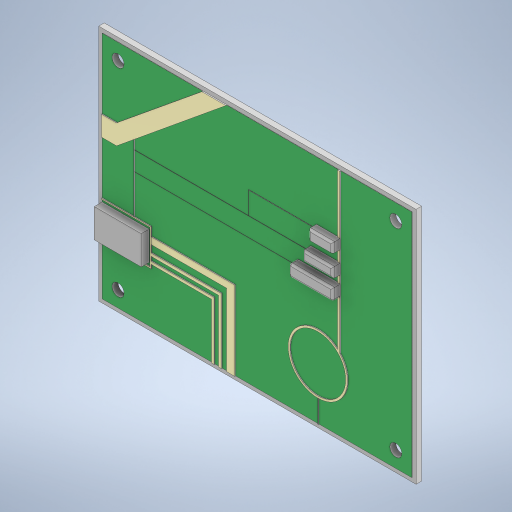
# Autodesk Inventor part: Board
Saved by Autodesk Inventor 2023 (Build 270158000, 158)
## iProperties
Created: 2022-11-08
Part Number: Board
Material: Generic
Document SubType Name: Modeling
Designer: 223076749
Density: 1 g/cm^3
Appearance: Default
Author: 223076749
Autodesk Inventor part; units mm, degrees
ref_plane "YZ Plane" through (0, 0, 0) normal (1, 0, 0) x (0, 1, 0)
ref_plane "XZ Plane" through (0, 0, 0) normal (0, 1, 0) x (-1, 0, 0)
ref_plane "XY Plane" through (0, 0, 0) normal (0, 0, 1) x (1, 0, 0)
sketch "Sketch1" plane through (0, 0, 0) normal (0, 0, 1) x (1, 0, 0)
  line L0 (0, 0) -> (203.2, 0)
  line L1 (203.2, 0) -> (203.2, 152.4)
  line L2 (203.2, 152.4) -> (0, 152.4)
  line L3 (0, 152.4) -> (0, 0)
  dimension "d0" = 203.2
  dimension "d1" = 152.4
  constraints: 8 end point, 2 parallel, 1 horizontal, 1 perpendicular
  measures "d0" distance of L2.end L1.end
  measures "d1" distance of L1.end L0.end
sketch "Sketch1 outline for Extrusion1" plane through (0, 0, 0) normal (0, 0, 1) x (1, 0, 0)
  line L0 (0, 0) -> (203.2, 0)
  line L1 (0, 152.4) -> (0, 0)
  line L2 (203.2, 152.4) -> (0, 152.4)
  line L3 (203.2, 0) -> (203.2, 152.4)
extrude "Extrusion1" add sketch "Sketch1 outline for Extrusion1" along normal blind 2.54
sketch "Sketch2" plane through (0, 0, 0) normal (0, 0, -1) x (-1, 0, 0)
  point P0 (0, 0)
sketch "Sketch4" plane through (0, 0, 2.54) normal (0, 0, 1) x (1, 0, 0)
  line L0 (0, 0) -> (203.2, 0) projected
  line L1 (101.6, 2.54) -> (200.66, 2.54)
  line L2 (200.66, 2.54) -> (200.66, 76.2)
  line L3 (2.54, 76.2) -> (2.54, 149.86)
  line L4 (0, 152.4) -> (0, 0) projected
  line L5 (2.54, 149.86) -> (101.6, 149.86)
  line L6 (203.2, 152.4) -> (0, 152.4) projected
  line L7 (200.66, 149.86) -> (101.6, 149.86)
  line L8 (203.2, 0) -> (203.2, 152.4) projected
  line L9 (200.66, 149.86) -> (200.66, 76.2)
  line L10 (2.54, 76.2) -> (2.54, 2.54)
  line L11 (2.54, 2.54) -> (101.6, 2.54)
  constraints: 16 end point, 4 perpendicular, 2 parallel, 2 point on line, 1 vertical
sketch "Sketch4 outline for Extrusion3" plane through (0, 0, 2.54) normal (0, 0, 1) x (1, 0, 0)
  line L0 (2.54, 76.2) -> (2.54, 2.54)
  line L1 (2.54, 149.86) -> (2.54, 76.2)
  line L2 (101.6, 149.86) -> (2.54, 149.86)
  line L3 (200.66, 149.86) -> (101.6, 149.86)
  line L4 (200.66, 76.2) -> (200.66, 149.86)
  line L5 (200.66, 2.54) -> (200.66, 76.2)
  line L6 (101.6, 2.54) -> (200.66, 2.54)
  line L7 (2.54, 2.54) -> (101.6, 2.54)
extrude "Extrusion3" add sketch "Sketch4 outline for Extrusion3" along normal blind 1.27
sketch "Sketch5" plane through (0, 0, 2.54) normal (0, 0, 1) x (1, 0, 0)
  line L0 (0, 0) -> (203.2, 0)
  line L1 (203.2, 0) -> (203.2, 152.4)
  line L2 (203.2, 152.4) -> (0, 152.4)
  line L3 (0, 152.4) -> (0, 0)
  line L4 (2.54, 149.86) -> (2.54, 2.54) projected
  line L5 (200.66, 149.86) -> (2.54, 149.86) projected
  line L6 (2.54, 2.54) -> (200.66, 2.54)
  line L7 (200.66, 2.54) -> (200.66, 149.86)
  line L8 (200.66, 149.86) -> (2.54, 149.86)
  line L9 (2.54, 149.86) -> (2.54, 2.54)
  constraints: 16 end point, 4 parallel, 2 horizontal, 2 perpendicular
sketch "Sketch5 outline for Extrusion4" plane through (0, 0, 2.54) normal (0, 0, 1) x (1, 0, 0)
  line L0 (0, 0) -> (203.2, 0)
  line L1 (0, 152.4) -> (0, 0)
  line L2 (203.2, 152.4) -> (0, 152.4)
  line L3 (203.2, 0) -> (203.2, 152.4)
extrude "Extrusion4" add sketch "Sketch5 outline for Extrusion4" along normal blind 1.016
sketch "Sketch6" plane through (0, 0, 3.81) normal (0, 0, 1) x (1, 0, 0)
  line L0 (0, 0) -> (12.7, 0)
  line L1 (12.7, 0) -> (12.7, 12.7)
  line L2 (12.7, 12.7) -> (0, 12.7)
  line L3 (0, 12.7) -> (0, 0)
  line L4 (203.2, 0) -> (190.5, 0)
  line L5 (190.5, 0) -> (190.5, 12.7)
  line L6 (190.5, 12.7) -> (203.2, 12.7)
  line L7 (203.2, 12.7) -> (203.2, 0)
  line L8 (203.2, 133.35) -> (203.2, 152.4)
  circle A0 centre (12.7, 12.7) radius 3.81
  circle A1 centre (190.5, 12.7) radius 3.81
  line L9 (203.2, 152.4) -> (0, 152.4) projected
  line L10 (0, 152.4) -> (12.7, 152.4)
  line L11 (12.7, 152.4) -> (12.7, 139.7)
  line L12 (12.7, 139.7) -> (0, 139.7)
  line L13 (0, 139.7) -> (0, 152.4)
  line L14 (203.2, 152.4) -> (190.5, 152.4)
  line L15 (190.5, 152.4) -> (190.5, 139.7)
  line L16 (190.5, 139.7) -> (203.2, 139.7)
  line L17 (203.2, 139.7) -> (203.2, 152.4)
  circle A2 centre (12.7, 139.7) radius 3.81
  circle A3 centre (190.5, 139.7) radius 3.81
  dimension "d18" = 12.7
  dimension "d19" = 12.7
  dimension "d21" = 12.7
  dimension "d22" = 12.7
  dimension "d28" = 7.62
  dimension "d29" = 7.62
  dimension "d30" = 12.7
  dimension "d31" = 12.7
  dimension "d32" = 12.7
  dimension "d33" = 12.7
  dimension "d34" = 7.62
  dimension "d35" = 7.62
  constraints: 34 end point, 8 parallel, 4 centre point, 4 coincident, 4 horizontal, 4 perpendicular
  measures "d18" distance of L2.end L1.end
  measures "d19" distance of L1.end L0.end
  measures "d21" distance of L5.end L6.end
  measures "d22" distance of L4.end L5.end
  measures "d28" diameter of A0
  measures "d29" diameter of A1
  measures "d30" distance of L11.end L12.end
  measures "d31" distance of L10.end L11.end
  measures "d32" distance of L16.end L15.end
  measures "d33" distance of L15.end L14.end
  measures "d34" diameter of A2
  measures "d35" diameter of A3
hole "Hole1" at (12.7, 139.7, 3.81) at (190.5, 139.7, 3.81) at (190.5, 12.7, 3.81) at (12.7, 12.7, 3.81) direction (0, 0, -1) diameter 7.62 end through all
sketch "Sketch7" plane through (0, 0, 3.81) normal (0, 0, 1) x (1, 0, 0)
  line L0 (2.54, 149.86) -> (2.54, 2.54)
  line L1 (2.54, 58.728997) -> (34.300412, 58.728997)
  line L2 (34.300412, 58.728997) -> (34.300412, 35.304324)
  line L3 (34.300412, 35.304324) -> (2.54, 35.304324)
  line L4 (2.54, 105.243705) -> (12.214291, 105.243705)
  line L5 (2.54, 98.870342) -> (12.214291, 98.870342)
  line L6 (12.214291, 98.870342) -> (73.177483, 148.650773)
  line L7 (12.214291, 92.520342) -> (2.54, 92.520342)
  line L8 (12.214291, 92.520342) -> (80.736552, 148.650773)
  line L9 (12.214291, 105.243705) -> (66.853266, 149.86)
  line L10 (200.66, 149.86) -> (2.54, 149.86)
  line L11 (73.177483, 148.650773) -> (74.658352, 149.86)
  line L12 (80.736552, 148.650773) -> (82.217421, 149.86)
  line L13 (2.54, 58.00717) -> (33.558011, 58.00717)
  line L14 (33.558011, 58.00717) -> (33.558011, 36.134305)
  line L15 (33.558011, 36.134305) -> (2.54, 36.134305)
  line L16 (2.54, 36.134305) -> (2.54, 58.00717)
  line L17 (2.54, 36.134305) -> (2.54, 35.304324)
  line L18 (2.54, 58.728997) -> (2.54, 58.00717)
  circle A0 centre (141.039906, 36.134305) radius 19.037306
  circle A1 centre (141.039906, 36.134305) radius 17.824973
  line L19 (138.373756, 98.870342) -> (158.864879, 98.870342)
  line L20 (158.864879, 98.870342) -> (158.864879, 92.520342)
  line L21 (158.864879, 92.520342) -> (138.373756, 92.520342)
  line L22 (138.373756, 92.520342) -> (138.373756, 98.870342)
  line L23 (138.373756, 112.547156) -> (158.864879, 112.547156)
  line L24 (158.864879, 112.547156) -> (158.864879, 106.496625)
  line L25 (158.864879, 106.496625) -> (138.373756, 106.496625)
  line L26 (138.373756, 106.496625) -> (138.373756, 112.547156)
  line L27 (158.864879, 87.286033) -> (151.567129, 87.286033)
  line L28 (151.567129, 87.286033) -> (151.567129, 83.13993)
  line L29 (151.567129, 83.13993) -> (158.864879, 83.13993)
  line L30 (158.864879, 83.13993) -> (158.864879, 87.286033)
  line L31 (155.216004, 149.86) -> (155.216004, 112.547156)
  line L32 (153.719902, 149.86) -> (153.719902, 112.547156)
  line L33 (153.719902, 106.496625) -> (153.719902, 98.870342)
  line L34 (155.216004, 106.496625) -> (155.216004, 98.870342)
  line L35 (153.719902, 92.520342) -> (153.719902, 87.286033)
  line L36 (155.216004, 92.520342) -> (155.216004, 87.286033)
  line L37 (153.719902, 149.86) -> (155.216004, 149.86)
  line L38 (200.66, 149.86) -> (2.54, 149.86)
  line L39 (153.719902, 112.547156) -> (155.216004, 112.547156)
  line L40 (2.54, 105.243705) -> (2.54, 92.520342)
  line L41 (66.853266, 149.86) -> (82.217421, 149.86)
  point P0 (0, 0)
  constraints: 78 end point, 27 point on line, 9 parallel, 9 perpendicular, 7 horizontal, 5 collinear, 2 centre point, 1 coincident, 1 midpoint, 1 vertical
sketch "Sketch7 outline for Extrusion6" plane through (0, 0, 3.81) normal (0, 0, 1) x (1, 0, 0)
  circle A0 centre (141.039906, 36.134305) radius 19.037306
  circle A1 centre (141.039906, 36.134305) radius 17.824973
  line L0 (34.300412, 35.304324) -> (34.300412, 58.728997)
  line L1 (2.54, 35.304324) -> (34.300412, 35.304324)
  line L2 (2.54, 36.134305) -> (2.54, 35.304324)
  line L3 (33.558011, 36.134305) -> (2.54, 36.134305)
  line L4 (33.558011, 58.00717) -> (33.558011, 36.134305)
  line L5 (2.54, 58.00717) -> (33.558011, 58.00717)
  line L6 (2.54, 58.728997) -> (2.54, 58.00717)
  line L7 (34.300412, 58.728997) -> (2.54, 58.728997)
  line L8 (82.217421, 149.86) -> (66.853266, 149.86)
  line L9 (80.736552, 148.650773) -> (82.217421, 149.86)
  line L10 (12.214291, 92.520342) -> (80.736552, 148.650773)
  line L11 (2.54, 92.520342) -> (12.214291, 92.520342)
  line L12 (2.54, 105.243705) -> (2.54, 92.520342)
  line L13 (12.214291, 105.243705) -> (2.54, 105.243705)
  line L14 (66.853266, 149.86) -> (12.214291, 105.243705)
  line L15 (155.216004, 87.286033) -> (155.216004, 92.520342)
  line L16 (153.719902, 87.286033) -> (155.216004, 87.286033)
  line L17 (153.719902, 92.520342) -> (153.719902, 87.286033)
  line L18 (155.216004, 92.520342) -> (153.719902, 92.520342)
  line L19 (155.216004, 98.870342) -> (155.216004, 106.496625)
  line L20 (153.719902, 98.870342) -> (155.216004, 98.870342)
  line L21 (153.719902, 106.496625) -> (153.719902, 98.870342)
  line L22 (155.216004, 106.496625) -> (153.719902, 106.496625)
  line L23 (153.719902, 149.86) -> (153.719902, 112.547156)
  line L24 (155.216004, 149.86) -> (153.719902, 149.86)
  line L25 (155.216004, 112.547156) -> (155.216004, 149.86)
  line L26 (153.719902, 112.547156) -> (155.216004, 112.547156)
extrude "Extrusion6" add sketch "Sketch7 outline for Extrusion6" along normal blind 0.508
sketch "Sketch9" plane through (0, 0, 3.81) normal (0, 0, 1) x (1, 0, 0)
  line L0 (155.216004, 112.547156) -> (155.216004, 149.86)
  line L1 (155.216004, 112.547156) -> (139.716798, 112.547156)
  line L2 (139.716798, 112.547156) -> (139.716798, 106.444154)
  line L3 (139.716798, 106.444154) -> (155.216004, 106.444154)
  line L4 (155.216004, 106.444154) -> (155.216004, 112.547156)
  line L5 (153.719902, 98.870342) -> (155.216004, 98.870342)
  line L6 (155.216004, 98.870342) -> (136.133648, 98.870342)
  line L7 (136.133648, 98.870342) -> (136.133648, 92.469871)
  line L8 (136.133648, 92.469871) -> (155.216004, 92.469871)
  line L9 (155.216004, 92.469871) -> (155.216004, 98.870342)
  line L10 (155.216004, 87.286033) -> (155.216004, 92.520342)
  line L11 (155.216004, 87.286033) -> (127.06376, 87.286033)
  line L12 (127.06376, 87.286033) -> (127.06376, 79.557955)
  line L13 (127.06376, 79.557955) -> (155.216004, 79.557955)
  line L14 (155.216004, 79.557955) -> (155.216004, 87.286033)
  line L15 (2.54, 58.00717) -> (2.54, 36.134305)
  line L16 (2.54, 56.327727) -> (32.618921, 56.327727)
  line L17 (32.618921, 56.327727) -> (32.618921, 37.841369)
  line L18 (32.618921, 37.841369) -> (2.54, 37.841369)
  line L19 (2.54, 37.841369) -> (2.54, 56.327727)
  point P0 (0, 0)
  constraints: 32 end point, 8 parallel, 4 horizontal, 4 perpendicular, 1 point on line
sketch "Sketch9 outline for Extrusion7" plane through (0, 0, 3.81) normal (0, 0, 1) x (1, 0, 0)
  line L0 (32.618921, 37.841369) -> (32.618921, 56.327727)
  line L1 (2.54, 37.841369) -> (32.618921, 37.841369)
  line L2 (2.54, 56.327727) -> (2.54, 37.841369)
  line L3 (32.618921, 56.327727) -> (2.54, 56.327727)
  line L4 (155.216004, 112.547156) -> (139.716798, 112.547156)
  line L5 (155.216004, 106.444154) -> (155.216004, 112.547156)
  line L6 (139.716798, 106.444154) -> (155.216004, 106.444154)
  line L7 (139.716798, 112.547156) -> (139.716798, 106.444154)
  line L8 (136.133648, 98.870342) -> (136.133648, 92.469871)
  line L9 (136.133648, 92.469871) -> (155.216004, 92.469871)
  line L10 (155.216004, 92.469871) -> (155.216004, 98.870342)
  line L11 (155.216004, 98.870342) -> (136.133648, 98.870342)
  line L12 (155.216004, 87.286033) -> (127.06376, 87.286033)
  line L13 (155.216004, 79.557955) -> (155.216004, 87.286033)
  line L14 (127.06376, 79.557955) -> (155.216004, 79.557955)
  line L15 (127.06376, 87.286033) -> (127.06376, 79.557955)
extrude "Extrusion7" add sketch "Sketch9 outline for Extrusion7" along normal blind 5.08
sketch "Sketch10" plane through (0, 0, 3.81) normal (0, 0, 1) x (1, 0, 0)
  line L0 (155.216004, 79.557955) -> (155.216004, 87.286033)
  line L1 (155.216004, 79.557955) -> (155.216004, 49.797318)
  line L2 (153.719902, 79.557955) -> (153.719902, 50.33419)
  circle A0 centre (141.039906, 36.134305) radius 19.037306
  line L3 (155.216004, 49.797318) -> (155.216004, 48.840889)
  line L4 (141.216863, 17.096999) -> (141.216863, 2.54)
  line L5 (2.54, 2.54) -> (200.66, 2.54)
  line L6 (141.039906, 17.227735) -> (141.039906, 2.54)
  line L7 (34.300412, 58.728997) -> (34.300412, 35.304324)
  line L8 (34.300412, 37.885472) -> (73.086359, 37.885472)
  line L9 (73.086359, 37.885472) -> (73.086359, 2.54)
  line L10 (34.300412, 39.683238) -> (74.644422, 39.683238)
  line L11 (74.644422, 39.683238) -> (74.644422, 2.54)
  line L12 (34.300412, 42.319961) -> (77.400997, 42.319961)
  line L13 (77.400997, 42.319961) -> (77.400997, 2.54)
  line L14 (34.300412, 44.237578) -> (79.318614, 44.237578)
  line L15 (79.318614, 44.237578) -> (79.318614, 2.54)
  line L16 (35.333277, 48.840889) -> (82.674443, 48.840889)
  line L17 (82.674443, 48.840889) -> (82.674443, 2.54)
  line L18 (35.333277, 48.840889) -> (33.558011, 48.840889)
  line L19 (33.558011, 36.134305) -> (33.558011, 58.00717)
  line L20 (34.445644, 53.226407) -> (87.828038, 53.226407)
  line L21 (87.828038, 53.226407) -> (87.828038, 2.54)
  line L22 (2.54, 58.728997) -> (34.300412, 58.728997)
  line L23 (23.211656, 58.728997) -> (23.211656, 101.528901)
  line L24 (80.736552, 148.650773) -> (12.214291, 92.520342)
  line L25 (23.211656, 58.728626) -> (23.211656, 101.528901)
  line L26 (23.325761, 58.728626) -> (23.325761, 101.622371)
  line L27 (155.216004, 48.840889) -> (153.719902, 50.33419)
  line L28 (127.06376, 79.557955) -> (155.216004, 79.557955)
  line L29 (153.719902, 79.557955) -> (155.216004, 79.557955)
  line L30 (141.216863, 2.54) -> (141.039906, 2.54)
  line L31 (141.039906, 17.096999) -> (141.216863, 17.096999)
  line L32 (82.674443, 2.54) -> (87.828038, 2.54)
  line L33 (79.318614, 2.54) -> (77.400997, 2.54)
  line L34 (74.644422, 2.54) -> (73.086359, 2.54)
  line L35 (34.445644, 48.840889) -> (34.445644, 53.226407)
  line L36 (34.300412, 42.319961) -> (34.300412, 44.237578)
  line L37 (34.300412, 37.885472) -> (34.300412, 39.683238)
  line L38 (23.211656, 58.728626) -> (23.325761, 58.728626)
  line L39 (23.211656, 101.528901) -> (23.325761, 101.622371)
  point P0 (0, 0)
  point P1 (23.325761, 58.728997)
  constraints: 66 end point, 9 horizontal, 7 vertical, 6 parallel, 6 point on line, 5 collinear, 4 perpendicular, 3 point on circle, 1 midpoint, 1 tangent, 8 other
sketch "Sketch10 outline for Extrusion8" plane through (0, 0, 3.81) normal (0, 0, 1) x (1, 0, 0)
  line L0 (23.325761, 58.728997) -> (23.325761, 101.622371)
  line L1 (23.211656, 58.728997) -> (23.325761, 58.728997)
  line L2 (23.211656, 101.528901) -> (23.211656, 58.728997)
  line L3 (23.325761, 101.622371) -> (23.211656, 101.528901)
  line L4 (74.644422, 2.54) -> (74.644422, 39.683238)
  line L5 (73.086359, 2.54) -> (74.644422, 2.54)
  line L6 (73.086359, 37.885472) -> (73.086359, 2.54)
  line L7 (34.300412, 37.885472) -> (73.086359, 37.885472)
  line L8 (34.300412, 39.683238) -> (34.300412, 37.885472)
  line L9 (74.644422, 39.683238) -> (34.300412, 39.683238)
  line L10 (79.318614, 2.54) -> (79.318614, 44.237578)
  line L11 (77.400997, 2.54) -> (79.318614, 2.54)
  line L12 (77.400997, 42.319961) -> (77.400997, 2.54)
  line L13 (34.300412, 42.319961) -> (77.400997, 42.319961)
  line L14 (34.300412, 44.237578) -> (34.300412, 42.319961)
  line L15 (79.318614, 44.237578) -> (34.300412, 44.237578)
  line L16 (34.445644, 48.840889) -> (82.674443, 48.840889)
  line L17 (82.674443, 48.840889) -> (82.674443, 2.54)
  line L18 (82.674443, 2.54) -> (87.828038, 2.54)
  line L19 (87.828038, 2.54) -> (87.828038, 53.226407)
  line L20 (87.828038, 53.226407) -> (34.445644, 53.226407)
  line L21 (34.445644, 53.226407) -> (34.445644, 48.840889)
  line L22 (141.216863, 17.096999) -> (141.039906, 17.096999)
  line L23 (141.216863, 2.54) -> (141.216863, 17.096999)
  line L24 (141.039906, 2.54) -> (141.216863, 2.54)
  line L25 (141.039906, 17.096999) -> (141.039906, 2.54)
  line L26 (153.719902, 50.33419) -> (155.216004, 48.840889)
  line L27 (155.216004, 48.840889) -> (155.216004, 79.557955)
  line L28 (155.216004, 79.557955) -> (153.719902, 79.557955)
  line L29 (153.719902, 79.557955) -> (153.719902, 50.33419)
extrude "Extrusion8" add sketch "Sketch10 outline for Extrusion8" along normal blind 0.508
fillet "Fillet1" radius 1.27 15 edges at (127.0638, 79.558, 6.35) (127.0638, 87.286, 6.35) (141.1399, 79.558, 8.89) (155.216, 79.558, 6.604) (141.1399, 87.286, 8.89) (155.216, 83.422, 8.89) (127.0638, 83.422, 8.89) (136.1336, 95.6701, 8.89) (145.6748, 92.4699, 8.89) (145.6748, 98.8703, 8.89) (155.216, 95.6701, 8.89) (139.7168, 109.4957, 8.89) (139.7168, 106.4442, 6.35) (155.216, 109.4957, 8.89) (147.4664, 112.5472, 8.89)
sketch "Sketch11" plane through (0, 0, 3.81) normal (0, 0, 1) x (1, 0, 0)
  line L0 (127.06376, 86.016033) -> (127.06376, 80.827955)
  line L1 (127.06376, 83.421994) -> (23.325761, 83.421994)
  line L2 (23.325761, 101.622371) -> (23.325761, 58.728997)
  line L3 (127.06376, 83.505558) -> (23.325761, 83.505558)
  line L4 (136.133648, 92.469871) -> (136.133648, 98.870342)
  line L5 (136.133648, 95.670107) -> (23.325761, 95.670107)
  line L6 (136.133648, 95.506171) -> (23.325761, 95.506171)
  line L7 (139.716798, 107.714154) -> (139.716798, 112.547156)
  line L8 (139.716798, 110.130655) -> (96.204133, 110.130655)
  line L9 (96.204133, 110.130655) -> (96.204133, 95.506171)
  line L10 (139.716798, 109.854619) -> (96.439333, 109.854619)
  line L11 (96.439333, 109.854619) -> (96.439333, 95.506171)
  line L12 (136.133648, 95.506171) -> (136.133648, 95.670107)
  line L13 (139.716798, 109.854619) -> (139.716798, 110.130655)
  line L14 (23.325761, 95.506171) -> (23.325761, 95.670107)
  line L15 (23.325761, 83.421994) -> (23.325761, 83.505558)
  line L16 (127.06376, 83.421994) -> (127.06376, 83.505558)
  point P0 (0, 0)
  point P1 (96.439333, 95.670107)
  point P2 (96.204133, 95.670107)
  constraints: 26 end point, 7 point on line, 5 collinear, 4 horizontal, 4 perpendicular, 3 midpoint
sketch "Sketch11 outline for Extrusion9" plane through (0, 0, 3.81) normal (0, 0, 1) x (1, 0, 0)
  line L0 (23.325761, 95.506171) -> (136.133648, 95.506171)
  line L1 (23.325761, 95.670107) -> (23.325761, 95.506171)
  line L2 (96.204133, 95.670107) -> (23.325761, 95.670107)
  line L3 (96.204133, 110.130655) -> (96.204133, 95.670107)
  line L4 (139.716798, 110.130655) -> (96.204133, 110.130655)
  line L5 (139.716798, 109.854619) -> (139.716798, 110.130655)
  line L6 (96.439333, 109.854619) -> (139.716798, 109.854619)
  line L7 (96.439333, 95.670107) -> (96.439333, 109.854619)
  line L8 (136.133648, 95.670107) -> (96.439333, 95.670107)
  line L9 (136.133648, 95.506171) -> (136.133648, 95.670107)
  line L10 (127.06376, 83.505558) -> (23.325761, 83.505558)
  line L11 (127.06376, 83.421994) -> (127.06376, 83.505558)
  line L12 (23.325761, 83.421994) -> (127.06376, 83.421994)
  line L13 (23.325761, 83.505558) -> (23.325761, 83.421994)
extrude "Extrusion9" add sketch "Sketch11 outline for Extrusion9" along normal blind 0.127
body "Solid1"
